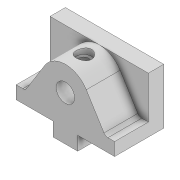
# Autodesk Inventor part: third
Saved by Autodesk Inventor 2020 (Build 240168000, 168)
## iProperties
Created: 2021-12-09
Part Number: third
Material: Generic
Document SubType Name: Modeling
Designer: NIKHIL VINOD
Density: 1 g/cm^3
Appearance: Default
Author: NIKHIL VINOD
Autodesk Inventor part; units mm, degrees
ref_plane "YZ Plane" through (0, 0, 0) normal (1, 0, 0) x (0, 1, 0)
ref_plane "XZ Plane" through (0, 0, 0) normal (0, 1, 0) x (-1, 0, 0)
ref_plane "XY Plane" through (0, 0, 0) normal (0, 0, 1) x (1, 0, 0)
sketch "Sketch1" plane through (0, 0, 0) normal (0, 0, 1) x (1, 0, 0)
  line L0 (64, 0) -> (64, 36)
  line L1 (64, 36) -> (0, 36)
  line L2 (0, 36) -> (0, 0)
  line L3 (40, 0) -> (40, -9)
  line L4 (40, -9) -> (24, -9)
  line L5 (24, -9) -> (24, 0)
  line L6 (0, 0) -> (24, 0)
  line L7 (40, 0) -> (64, 0)
  dimension "d0" = 64
  dimension "d1" = 36
  dimension "d2" = 16
  dimension "d3" = 9
  dimension "d4" = 24
  constraints: 16 end point, 4 parallel, 2 horizontal, 2 perpendicular
  measures "d0" distance of L1.end L0.end
  measures "d1" distance of L0.end L0.start
  measures "d2" distance of L3.end L4.end
  measures "d3" distance of L3.start L3.end
  measures "d4" distance between parallel lines of L5 L2
extrude "Extrusion1" add sketch "Sketch1" along normal blind 32
sketch "Sketch2" plane through (0, 0, 32) normal (0, 0, 1) x (1, 0, 0)
  circle A0 centre (32, 20) radius 6
  line L0 (0, 36) -> (0, 0) projected
  line L1 (40, 0) -> (64, 0) projected
  arc A1 (45.5949, 28.4368) -> (18.4051, 28.4368) centre (32, 20) ccw
  line L2 (0, 8.4474) -> (4.331, 8.4474)
  line L3 (6.8801, 9.8655) -> (18.4051, 28.4368)
  line L4 (64, 0) -> (64, 36) projected
  line L5 (64, 8.4474) -> (59.669, 8.4474)
  line L6 (57.1199, 9.8655) -> (45.5949, 28.4368)
  arc A2 (4.331, 8.4474) -> (6.8801, 9.8655) centre (4.331, 11.4474) ccw
  arc A3 (57.1199, 9.8655) -> (59.669, 8.4474) centre (59.669, 11.4474) ccw
  line L7 (0, 8.4474) -> (0, 36)
  line L8 (64, 36) -> (0, 36) projected
  line L9 (0, 36) -> (64, 36)
  line L10 (64, 36) -> (64, 8.4474)
  point P0 (6, 8.4474)
  point P1 (58, 8.4474)
  point P2 (32, 36)
  dimension "d7" = 12
  dimension "d8" = 32
  dimension "d9" = 20
  dimension "d10" = 6
  dimension "d11" = 32
  dimension "d12" = 6
  dimension "d13" = 3
  constraints: 14 end point, 8 point on line, 6 point on circle, 6 tangent, 4 centre point, 1 coincident, 1 collinear, 1 equal radius, 1 horizontal, 1 perpendicular, 1 vertical
  measures "d7" diameter of A0
  measures "d8" distance from line of L0 A0.centre
  measures "d9" distance from line of L1 A0.centre
  measures "d10" distance of L2.start point (6, 8.447)
  measures "d11" diameter of A1
  measures "d12" distance of L5.start point (58, 8.447)
  measures "d13" radius of A2
extrude "Extrusion2" cut sketch "Sketch2" against normal blind 22 contours L8 A1 L3 A2 L2 L0 | L8 L4 L5 A3 L6 A1
sketch "Sketch3" plane through (0, 0, 32) normal (0, 0, 1) x (1, 0, 0)
  circle A0 centre (32, 20) radius 6
  line L0 (0, 8.4474) -> (0, 36) projected
  line L1 (40, 0) -> (64, 0) projected
  point P0 (0, 0)
  dimension "d16" = 12
  dimension "d17" = 32
  dimension "d18" = 20
  constraints: 1 centre point
  measures "d16" diameter of A0
  measures "d17" distance from line of L0 A0.centre
  measures "d18" distance from line of L1 A0.centre
extrude "Extrusion3" cut sketch "Sketch3" against normal blind 24
sketch "Sketch4" plane through (0, 36, 0) normal (0, 1, 0) x (1, 0, 0)
  circle A0 centre (32, -20) radius 3
  line L0 (18.4051, -32) -> (45.5949, -32) projected
  line L1 (0, -32) -> (0, -10) projected
  point P0 (0, 0)
  dimension "d21" = 6
  dimension "d22" = 12
  dimension "d23" = 32
  constraints: 1 centre point
  measures "d21" diameter of A0
  measures "d22" distance from line of L0 A0.centre
  measures "d23" distance from line of L1 A0.centre
extrude "Extrusion4" cut sketch "Sketch4" against normal blind 16
sketch "Sketch5" plane through (0, 36, 0) normal (0, 1, 0) x (1, 0, 0)
  circle A0 centre (32, -20) radius 5
  line L0 (18.4051, -32) -> (45.5949, -32) projected
  line L1 (0, -32) -> (0, -10) projected
  point P0 (0, 0)
  dimension "d26" = 10
  dimension "d27" = 12
  dimension "d28" = 32
  constraints: 1 centre point
  measures "d26" diameter of A0
  measures "d27" distance from line of L0 A0.centre
  measures "d28" distance from line of L1 A0.centre
extrude "Extrusion5" cut sketch "Sketch5" against normal blind 4
sketch "Sketch6" plane through (24, -9, 0) normal (0, -1, 0) x (1, 0, 0)
  circle A0 centre (8, 24) radius 3
  circle A1 centre (8, 8) radius 3
  line L0 (0, 32) -> (16, 32) projected
  point P0 (-24, 0)
  dimension "d31" = 6
  dimension "d32" = 6
  dimension "d33" = 8
  dimension "d34" = 16
  constraints: 2 centre point
  measures "d31" diameter of A0
  measures "d32" diameter of A1
  measures "d33" distance from line of L0 A0.centre
  measures "d34" distance of A1.centre A0.centre
extrude "Extrusion6" cut sketch "Sketch6" against normal blind 16
body "Solid1"
